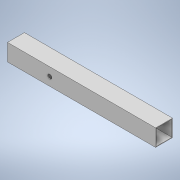
# Autodesk Inventor part: CatapultArm
Saved by Autodesk Inventor 2022.2 (Build 262287000, 287)
## iProperties
Created: 2022-01-16
Part Number: CatapultArm
Material: Generic
Document SubType Name: Modeling
Designer: robst
Density: 1 g/cm^3
Appearance: Default
Author: robst
Autodesk Inventor part; units mm, degrees
ref_plane "YZ Plane" through (0, 0, 0) normal (1, 0, 0) x (0, 1, 0)
ref_plane "XZ Plane" through (0, 0, 0) normal (0, 1, 0) x (-1, 0, 0)
ref_plane "XY Plane" through (0, 0, 0) normal (0, 0, 1) x (1, 0, 0)
sketch "Sketch2" plane through (0, 0, 0) normal (0, 0, 1) x (1, 0, 0)
  circle A0 centre (0, 0) radius 12.7
  line L0 (12.7, 0) -> (635, 0)
  line L1 (635, 0) -> (635, 50.8)
  line L2 (635, 50.8) -> (0, 50.8)
  line L3 (0, 50.8) -> (0, 12.7)
  line L4 (635, 0) -> (635, -50.8)
  line L5 (635, -50.8) -> (0, -50.8)
  line L6 (0, -50.8) -> (0, -12.7)
  line L7 (-12.7, 0) -> (-254, 0)
  line L8 (-254, 0) -> (-254, 50.8)
  line L9 (-254, 50.8) -> (0, 50.8)
  line L10 (0, 50.8) -> (0, 12.7)
  line L11 (0, -50.8) -> (0, -12.7)
  line L12 (-254, 0) -> (-254, -50.8)
  line L13 (-254, -50.8) -> (0, -50.8)
  dimension "d0" = 25.4
  dimension "d1" = 50.8
  dimension "d2" = 635
  dimension "d3" = 254
  constraints: 28 end point, 6 symmetric about line, 4 parallel, 3 point on circle, 2 horizontal, 2 perpendicular, 1 centre point, 1 coincident, 1 point on line
  measures "d0" diameter of A0
  measures "d1" distance of L0.end L1.end
  measures "d2" distance of L1.end L2.end
  measures "d3" distance of L8.end L9.end
extrude "Extrusion1" add sketch "Sketch2" along normal mid plane 101.6 contours L0 L4 L5 L6 A0 | A0 L3 L2 L1 L0 | A0 L7 L8 L9 L3 | L6 L13 L12 L7 A0
sketch "Sketch3" plane through (0, 0, 0) normal (1, 0, 0) x (0, 1, 0)
  line L0 (50.8, -50.8) -> (50.8, 50.8) projected
  line L1 (-50.8, -50.8) -> (50.8, -50.8) projected
  line L2 (50.8, 50.8) -> (-50.8, 50.8) projected
  line L3 (-50.8, -50.8) -> (-50.8, 50.8) projected
  line L4 (-50.8, 50.8) -> (-50.8, -50.8)
  line L5 (-50.8, -50.8) -> (50.8, -50.8)
  line L6 (50.8, -50.8) -> (50.8, 50.8)
  line L7 (50.8, 50.8) -> (-50.8, 50.8)
  line L8 (-50.8, 50.8) -> (50.8, -50.8) construction
  line L9 (-50.8, -50.8) -> (50.8, 50.8) construction
  line L10 (-47.625, 47.625) -> (-47.625, -47.625)
  line L11 (-47.625, -47.625) -> (47.625, -47.625)
  line L12 (47.625, -47.625) -> (47.625, 47.625)
  line L13 (47.625, 47.625) -> (-47.625, 47.625)
  line L14 (-47.625, 47.625) -> (47.625, -47.625) construction
  line L15 (-47.625, -47.625) -> (47.625, 47.625) construction
  line L16 (-12.7, 50.8) -> (-12.7, -50.8) projected
  point P0 (0, 0)
  point P1 (-12.7, 47.625)
  point P2 (-12.7, -47.625)
  dimension "d6" = 3.175
  dimension "d7" = 3.175
  constraints: 24 end point, 5 parallel, 4 midpoint, 2 perpendicular
  measures "d6" distance between parallel lines of L12 L0
  measures "d7" distance between parallel lines of L2 L13
extrude "Extrusion3" cut sketch "Sketch3" along normal through all both and the other way through all contours L16 L13 L12 L11 | L11 L10 L13 L16
equation "\"d2\" = longDistanceFromHole"
equation "\"d3\" = shortDistanceFromHole"
equation "\"materialWidth\" = 101.6"
equation "\"shortDistanceFromHole\" = 254"
equation "\"longDistanceFromHole\" = 635"
body "Solid1"
